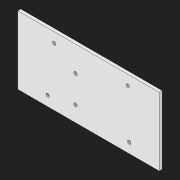
# Autodesk Inventor part: BP007
Saved by Autodesk Inventor 2017 SP1 (Build 210196100, 196)
## iProperties
Created: 2018-03-09
Part Number: BP007
Material: ABS Plastic
Document SubType Name: Modeling
Designer: Zach
Density: 1.06 g/cm^3
Appearance: CR White
Author: Zach
Autodesk Inventor part; units mm, degrees
ref_plane "YZ Plane" through (0, 0, 0) normal (1, 0, 0) x (0, 1, 0)
ref_plane "XZ Plane" through (0, 0, 0) normal (0, 1, 0) x (-1, 0, 0)
ref_plane "XY Plane" through (0, 0, 0) normal (0, 0, 1) x (1, 0, 0)
sketch "Sketch1" plane through (0, 0, 0) normal (0, 0, 1) x (1, 0, 0)
  circle A0 centre (6.5, 48.4) radius 1.7
  circle A1 centre (82, 0) radius 1.7
  circle A2 centre (0, 0) radius 1.7
  circle A3 centre (28, 5.5) radius 1.7
  circle A4 centre (28, 32.9) radius 1.7
  line L0 (0, 0) -> (82, 0) construction
  circle A5 centre (80.5, 48.4) radius 1.7
  line L1 (82, 0) -> (80.5, 48.4) construction
  line L2 (80.5, 48.4) -> (6.5, 48.4) construction
  line L3 (6.5, 48.4) -> (0, 0) construction
  line L4 (28, 5.5) -> (28, 32.9) construction
  line L5 (-30, 58.4) -> (112, 58.4)
  line L6 (112, 58.4) -> (112, -10)
  line L7 (112, -10) -> (-30, -10)
  line L8 (-30, -10) -> (-30, 58.4)
  dimension "d0" = 82
  dimension "d1" = 48.4
  dimension "d2" = 48.4
  dimension "d3" = 74
  dimension "d4" = 27.4
  dimension "d5" = 5.5
  dimension "d6" = 28
  dimension "d7" = 6.5
  dimension "d10" = 3.4
  dimension "d11" = 3.4
  dimension "d12" = 3.4
  dimension "d13" = 3.4
  dimension "d15" = 3.4
  dimension "d16" = 3.4
  dimension "d17" = 10
  dimension "d18" = 30
  dimension "d19" = 10
  dimension "d20" = 30
  constraints: 18 end point, 6 centre point, 2 horizontal, 2 parallel, 1 coincident, 1 perpendicular, 1 vertical
  measures "d0" distance of L0.start L0.end
  measures "d1" vertical distance of L0.end L1.end
  measures "d2" vertical distance of L2.end L0.start
  measures "d3" distance of L1.end L2.end
  measures "d4" distance of L4.start L4.end
  measures "d5" distance from line of L0 L4.start
  measures "d6" distance from line of L0.start L4
  measures "d7" horizontal distance of L0.start L2.end
  measures "d10" diameter of A0
  measures "d11" diameter of A2
  measures "d12" diameter of A3
  measures "d13" diameter of A4
  measures "d15" diameter of A1
  measures "d16" diameter of A5
  measures "d17" distance from line of L7 L0.start
  measures "d18" distance from line of point (0, 0) L8
  measures "d19" distance from line of L5 L1.end
  measures "d20" distance from line of L0.end L6
extrude "Extrusion1" add sketch "Sketch1" along normal blind 3
body "Solid1"
